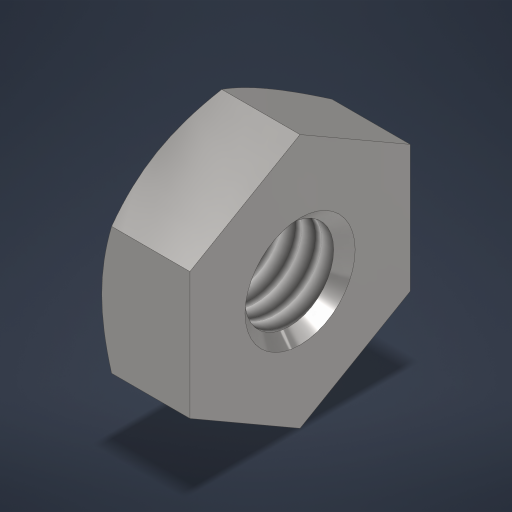
# Autodesk Inventor part: SLBNR2.5
Saved by Autodesk Inventor 2023.3 (Build 273359000, 359)
## iProperties
Created: 2023-10-29
Part Number: SLBNR2.5
Material: 스테인리스스틸, 감마철
Catalog Web Link: www.cadenas.de
Description: LBNR, LBNL, SLBNR, SLBNL, KNTR, KNTL, SKNTR-Nuts
Vendor: MISUMI
Document SubType Name: Modeling
Designer: psAdmin
Manufacturer: MISUMI
Mass: 0.291162 g
Surface Area: 0.815607 cm^2
Volume: 0.0363952 cm^3
Density: 8 g/cm^3
Appearance: 반연마
Category: PARTsolutions
Company: MISUMI
PSOL_IDENT_0: {$CADENAS_DATA/23d-libs/misumi/metric/27_screws_nuts/slbnl.prj},204 {VTYP=3D},{NB=SLBNR2.5},{LINA=SL
PSOL_IDENT_1: BNR2.5},{NN=LBNR, LBNL, SLBNR, SLBNL, KNTR, KNTL, SKNTR},{DATE=03.06.2021 03:35:45},{GEOMDATE=05.11.
PSOL_IDENT_2: 2010 00:00:00},{VERSION=},{LINEID=130},{WBVAR=TRS,MAT,CS},{WBNUMERIC=}  {NB=SLBNR2.5},{LINA=SLBNR2.5
PSOL_IDENT_3: },{KT=DUMMY},{PN=SLBNR2.5},{TS=LBN},{TRS=R},{MAT=S},{ST=-},{CS=1},{M1=2.5},{M=2.5},{P=0.45},{B=5.0},
PSOL_IDENT_4: {EE=5.8},{T=2.0},{T1=0.0},{TFX=2.0},{T1FX=1.6},{CALG='1','JIS Class 1'},{TRSALG= 'R', 'Right-Hand Th
PSOL_IDENT_5: read' },{MATALG= '', 'SWCH Carbon Steel', 'S', '304 Stainless Steel' }
NB: SLBNR2.5
NN: LBNR, LBNL, SLBNR, SLBNL, KNTR, KNTL, SKNTR
NT: Nuts
NBSYN: $PN.
LINA: SLBNR2.5
CATALOG: Misumi
PN: SLBNR2.5
TRS: Right-Hand Thread
MAT: 304 Stainless Steel Equivalent
ST: -
CS: JIS Class 1
M1: 2.5
P: 0.45
B: 5
EE: 5.8
T: 2
T1: 0
SUPPLIER: MISUMI
ARTICLENO: SLBNR2.5
BOMINFO: SLBNR2.5
CREATOR: CADENAS GmbH
Title: SLBNR2.5
Author: Cadenas PARTsolutions
Comments: Nuts
Autodesk Inventor part; units mm, degrees
sketch "Sketch_1" plane through (0, 0, 0) normal (0, 0, 1) x (1, 0, 0)
  line L0 (1, 0) -> (-1, 0)
  line L1 (-1, 0) -> (-1, 2.5)
  line L2 (-1, 2.5) -> (-0.7691, 2.9)
  line L3 (-0.7691, 2.9) -> (1, 2.9)
  line L4 (1, 2.9) -> (1, 0)
  line L5 (1, 0) -> (-1, 0)
  constraints: 12 end point
revolve "Revolution1" add sketch "Sketch_1" angle 360 about axis through (1, 0, 0) along (1, 0, 0)
sketch "Sketch_2" plane through (0, 0, 0) normal (0, 0, 1) x (1, 0, 0)
  line L0 (1, 0) -> (-1, 0)
  line L1 (-1, 0) -> (-1, 1.25)
  line L2 (-1, 1.25) -> (-0.7565, 1.0065)
  line L3 (-0.7565, 1.0065) -> (0.7565, 1.0065)
  line L4 (0.7565, 1.0065) -> (1, 1.25)
  line L5 (1, 1.25) -> (1, 0)
  line L6 (1, 0) -> (-1, 0)
  constraints: 14 end point
revolve "Revolution2" cut sketch "Sketch_2" angle 360 about axis through (1, 0, 0) along (1, 0, 0)
thread "Thread1" size "M2.5x0.45" class "6H" standard "ISO Metric profile" full length
sketch "Sketch_3" plane through (0, 0, 0) normal (1, 0, 0) x (0, 1, 0)
  line L0 (-5, 5) -> (-5, -5)
  line L1 (-5, -5) -> (5, -5)
  line L2 (5, -5) -> (5, 5)
  line L3 (5, 5) -> (-5, 5)
  line L4 (-1.4434, 2.5) -> (-2.8868, 0)
  line L5 (-2.8868, 0) -> (-1.4434, -2.5)
  line L6 (-1.4434, -2.5) -> (1.4434, -2.5)
  line L7 (1.4434, -2.5) -> (2.8868, 0)
  line L8 (2.8868, 0) -> (1.4434, 2.5)
  line L9 (1.4434, 2.5) -> (-1.4434, 2.5)
  constraints: 20 end point
extrude "Extrusion1" cut sketch "Sketch_3" along normal mid plane 2
ref_plane "cp_XY" through (1, 0, 0) normal (1, 0, 0) x (0, 0, -1)
ref_plane "cp_YZ" through (1, 0, 0) normal (0, 0, -1) x (0, 1, 0)
ref_plane "cp_ZX" through (1, 0, 0) normal (0, 1, 0) x (1, 0, 0)
ref_plane "nut_to_screw_XY" through (0, 0, 0) normal (1, 0, 0) x (0, 0, -1)
ref_plane "nut_to_screw_YZ" through (0, 0, 0) normal (0, 0, -1) x (0, 1, 0)
ref_plane "nut_to_screw_ZX" through (0, 0, 0) normal (0, 1, 0) x (1, 0, 0)
body "Solid1"
